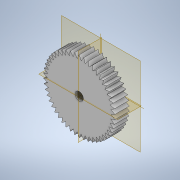
# Autodesk Inventor part: Zahnrad
Saved by Autodesk Inventor 2022 (Build 260153000, 153)
## iProperties
Created: 2022-05-06
Part Number: Zahnrad
Material: Generisch
Document SubType Name: Modeling
Designer: 123St
Density: 1 g/cm^3
Appearance: Vorgabe
Author: 123St
Autodesk Inventor part; units mm, degrees
sketch "Skizze1" plane through (0, 0, 0) normal (0, 0, 1) x (1, 0, 0)
  circle A0 centre (0, 0) radius 2.95
  circle A1 centre (0, 0) radius 5
  dimension "d0" = 5.9
  dimension "d1" = 10
  constraints: 2 centre point, 2 coincident
  measures "d0" diameter of A0
  measures "d1" diameter of A1
extrude "Extrusion1" add sketch "Skizze1" along normal blind 3
sketch "Skizze2" plane through (0, 0, 3) normal (0, 0, 1) x (1, 0, 0)
  circle A0 centre (0, 0) radius 15
  circle A1 centre (0, 0) radius 1.75
  dimension "d4" = 30
  dimension "d5" = 3.5
  constraints: 2 centre point, 2 coincident
  measures "d4" diameter of A0
  measures "d5" diameter of A1
extrude "Extrusion2" add sketch "Skizze2" along normal blind 6
sketch "Skizze3" plane through (0, 0, 9) normal (0, 0, 1) x (1, 0, 0)
  circle A0 centre (0, 0) radius 15 projected
  line L0 (0, 15) -> (-0.95, 13)
  line L1 (0, 15) -> (0.95, 13)
  line L2 (0, 21) -> (0, -21) projected
  line L3 (1.88, 14.8817) -> (0.6868, 13.0166)
  line L4 (1.88, 14.8817) -> (2.5718, 12.7784)
  line L5 (3.7303, 14.5287) -> (2.3128, 12.8278)
  line L6 (3.7303, 14.5287) -> (4.1531, 12.3553)
  line L7 (5.5219, 13.9466) -> (3.9023, 12.4368)
  line L8 (5.5219, 13.9466) -> (5.6689, 11.7374)
  line L9 (7.2263, 13.1446) -> (5.4303, 11.8497)
  line L10 (7.2263, 13.1446) -> (7.0953, 10.9343)
  line L11 (8.8168, 12.1353) -> (6.8726, 11.0756)
  line L12 (8.8168, 12.1353) -> (8.4098, 9.9588)
  line L13 (10.2682, 10.9345) -> (8.2066, 10.1269)
  line L14 (10.2682, 10.9345) -> (9.5916, 8.8263)
  line L15 (11.5577, 9.5614) -> (9.4111, 9.0185)
  line L16 (11.5577, 9.5614) -> (10.6222, 7.5545)
  line L17 (12.6649, 8.0374) -> (10.4672, 7.7679)
  line L18 (12.6649, 8.0374) -> (11.4853, 6.1636)
  line L19 (13.5724, 6.3867) -> (11.3583, 6.3947)
  line L20 (13.5724, 6.3867) -> (12.1672, 4.6755)
  line L21 (14.2658, 4.6353) -> (12.0702, 4.9207)
  line L22 (14.2658, 4.6353) -> (12.6573, 3.1137)
  line L23 (14.7343, 2.8107) -> (12.5917, 3.3691)
  line L24 (14.7343, 2.8107) -> (12.9477, 1.5028)
  line L25 (14.9704, 0.9419) -> (12.9147, 1.7644)
  line L26 (14.9704, 0.9419) -> (13.034, -0.1318)
  line L27 (14.9704, -0.9419) -> (13.034, 0.1318)
  line L28 (14.9704, -0.9419) -> (12.9147, -1.7644)
  line L29 (14.7343, -2.8107) -> (12.9477, -1.5028)
  line L30 (14.7343, -2.8107) -> (12.5917, -3.3691)
  line L31 (14.2658, -4.6353) -> (12.6573, -3.1137)
  line L32 (14.2658, -4.6353) -> (12.0702, -4.9207)
  line L33 (13.5724, -6.3867) -> (12.1672, -4.6755)
  line L34 (13.5724, -6.3867) -> (11.3583, -6.3947)
  line L35 (12.6649, -8.0374) -> (11.4853, -6.1636)
  line L36 (12.6649, -8.0374) -> (10.4672, -7.7679)
  line L37 (11.5577, -9.5614) -> (10.6222, -7.5545)
  line L38 (11.5577, -9.5614) -> (9.4111, -9.0185)
  line L39 (10.2682, -10.9345) -> (9.5916, -8.8263)
  line L40 (10.2682, -10.9345) -> (8.2066, -10.1269)
  line L41 (8.8168, -12.1353) -> (8.4098, -9.9588)
  line L42 (8.8168, -12.1353) -> (6.8726, -11.0756)
  line L43 (7.2263, -13.1446) -> (7.0953, -10.9343)
  line L44 (7.2263, -13.1446) -> (5.4303, -11.8497)
  line L45 (5.5219, -13.9466) -> (5.6689, -11.7374)
  line L46 (5.5219, -13.9466) -> (3.9023, -12.4368)
  line L47 (3.7303, -14.5287) -> (4.1531, -12.3553)
  line L48 (3.7303, -14.5287) -> (2.3128, -12.8278)
  line L49 (1.88, -14.8817) -> (2.5718, -12.7784)
  line L50 (1.88, -14.8817) -> (0.6868, -13.0166)
  line L51 (0, -15) -> (0.95, -13)
  line L52 (0, -15) -> (-0.95, -13)
  line L53 (-1.88, -14.8817) -> (-0.6868, -13.0166)
  line L54 (-1.88, -14.8817) -> (-2.5718, -12.7784)
  line L55 (-3.7303, -14.5287) -> (-2.3128, -12.8278)
  line L56 (-3.7303, -14.5287) -> (-4.1531, -12.3553)
  line L57 (-5.5219, -13.9466) -> (-3.9023, -12.4368)
  line L58 (-5.5219, -13.9466) -> (-5.6689, -11.7374)
  line L59 (-7.2263, -13.1446) -> (-5.4303, -11.8497)
  line L60 (-7.2263, -13.1446) -> (-7.0953, -10.9343)
  line L61 (-8.8168, -12.1353) -> (-6.8726, -11.0756)
  line L62 (-8.8168, -12.1353) -> (-8.4098, -9.9588)
  line L63 (-10.2682, -10.9345) -> (-8.2066, -10.1269)
  line L64 (-10.2682, -10.9345) -> (-9.5916, -8.8263)
  line L65 (-11.5577, -9.5614) -> (-9.4111, -9.0185)
  line L66 (-11.5577, -9.5614) -> (-10.6222, -7.5545)
  line L67 (-12.6649, -8.0374) -> (-10.4672, -7.7679)
  line L68 (-12.6649, -8.0374) -> (-11.4853, -6.1636)
  line L69 (-13.5724, -6.3867) -> (-11.3583, -6.3947)
  line L70 (-13.5724, -6.3867) -> (-12.1672, -4.6755)
  line L71 (-14.2658, -4.6353) -> (-12.0702, -4.9207)
  line L72 (-14.2658, -4.6353) -> (-12.6573, -3.1137)
  line L73 (-14.7343, -2.8107) -> (-12.5917, -3.3691)
  line L74 (-14.7343, -2.8107) -> (-12.9477, -1.5028)
  line L75 (-14.9704, -0.9419) -> (-12.9147, -1.7644)
  line L76 (-14.9704, -0.9419) -> (-13.034, 0.1318)
  line L77 (-14.9704, 0.9419) -> (-13.034, -0.1318)
  line L78 (-14.9704, 0.9419) -> (-12.9147, 1.7644)
  line L79 (-14.7343, 2.8107) -> (-12.9477, 1.5028)
  line L80 (-14.7343, 2.8107) -> (-12.5917, 3.3691)
  line L81 (-14.2658, 4.6353) -> (-12.6573, 3.1137)
  line L82 (-14.2658, 4.6353) -> (-12.0702, 4.9207)
  line L83 (-13.5724, 6.3867) -> (-12.1672, 4.6755)
  line L84 (-13.5724, 6.3867) -> (-11.3583, 6.3947)
  line L85 (-12.6649, 8.0374) -> (-11.4853, 6.1636)
  line L86 (-12.6649, 8.0374) -> (-10.4672, 7.7679)
  line L87 (-11.5577, 9.5614) -> (-10.6222, 7.5545)
  line L88 (-11.5577, 9.5614) -> (-9.4111, 9.0185)
  line L89 (-10.2682, 10.9345) -> (-9.5916, 8.8263)
  line L90 (-10.2682, 10.9345) -> (-8.2066, 10.1269)
  line L91 (-8.8168, 12.1353) -> (-8.4098, 9.9588)
  line L92 (-8.8168, 12.1353) -> (-6.8726, 11.0756)
  line L93 (-7.2263, 13.1446) -> (-7.0953, 10.9343)
  line L94 (-7.2263, 13.1446) -> (-5.4303, 11.8497)
  line L95 (-5.5219, 13.9466) -> (-5.6689, 11.7374)
  line L96 (-5.5219, 13.9466) -> (-3.9023, 12.4368)
  circle A1 centre (0, 0) radius 15
  line L97 (-3.7303, 14.5287) -> (-4.1531, 12.3553)
  line L98 (-3.7303, 14.5287) -> (-2.3128, 12.8278)
  line L99 (-1.88, 14.8817) -> (-2.5718, 12.7784)
  line L100 (-1.88, 14.8817) -> (-0.6868, 13.0166)
  point P0 (-4.1012, 12.6222)
  point P1 (-3.7303, 14.5287)
  point P2 (-3.7303, 14.5287)
  point P3 (-5.5219, 13.9466)
  point P4 (-5.6509, 12.0087)
  point P5 (-7.2263, 13.1446)
  point P6 (-7.2263, 13.1446)
  point P7 (-7.1114, 11.2057)
  point P8 (-8.4598, 10.2261)
  point P9 (-10.2682, 10.9345)
  point P10 (-10.2682, 10.9345)
  point P11 (-9.6747, 9.0852)
  point P12 (-11.5577, 9.5614)
  point P13 (-10.7371, 7.801)
  point P14 (-12.6649, 8.0374)
  point P15 (-12.6649, 8.0374)
  point P16 (-11.6302, 6.3937)
  point P17 (-12.3398, 4.8857)
  point P18 (-14.2658, 4.6353)
  point P19 (-12.8548, 3.3006)
  point P20 (-13.1671, 1.6634)
  point P21 (-14.9704, 0.9419)
  point P22 (-14.9704, 0.9419)
  point P23 (-13.2718, 0)
  point P24 (-14.9704, -0.9419)
  point P25 (-14.9704, -0.9419)
  point P26 (-13.1671, -1.6634)
  point P27 (-14.7343, -2.8107)
  point P28 (-14.7343, -2.8107)
  point P29 (-12.8548, -3.3006)
  point P30 (-14.2658, -4.6353)
  point P31 (-12.3398, -4.8857)
  point P32 (-13.5724, -6.3867)
  point P33 (-11.6302, -6.3937)
  point P34 (-12.6649, -8.0374)
  point P35 (-10.7371, -7.801)
  point P36 (-9.6747, -9.0852)
  point P37 (-10.2682, -10.9345)
  point P38 (-10.2682, -10.9345)
  point P39 (-8.4598, -10.2261)
  point P40 (-8.8168, -12.1353)
  point P41 (-7.1114, -11.2057)
  point P42 (-7.2263, -13.1446)
  point P43 (-7.2263, -13.1446)
  point P44 (-5.6509, -12.0087)
  point P45 (-5.5219, -13.9466)
  point P46 (-5.5219, -13.9466)
  point P47 (-4.1012, -12.6222)
  point P48 (-3.7303, -14.5287)
  point P49 (-2.4869, -13.0367)
  point P50 (-1.88, -14.8817)
  point P51 (-1.88, -14.8817)
  point P52 (-0.8333, -13.2456)
  point P53 (0, -15)
  point P54 (0, -15)
  point P55 (0.8333, -13.2456)
  point P56 (1.88, -14.8817)
  point P57 (1.88, -14.8817)
  point P58 (2.4869, -13.0367)
  point P59 (3.7303, -14.5287)
  point P60 (3.7303, -14.5287)
  point P61 (4.1012, -12.6222)
  point P62 (5.5219, -13.9466)
  point P63 (5.6509, -12.0087)
  point P64 (7.2263, -13.1446)
  point P65 (7.2263, -13.1446)
  point P66 (7.1114, -11.2057)
  point P67 (8.8168, -12.1353)
  point P68 (8.4598, -10.2261)
  point P69 (10.2682, -10.9345)
  point P70 (9.6747, -9.0852)
  point P71 (11.5577, -9.5614)
  point P72 (10.7371, -7.801)
  point P73 (12.6649, -8.0374)
  point P74 (11.6302, -6.3937)
  point P75 (13.5724, -6.3867)
  point P76 (12.3398, -4.8857)
  point P77 (14.2658, -4.6353)
  point P78 (12.8548, -3.3006)
  point P79 (14.7343, -2.8107)
  point P80 (14.7343, -2.8107)
  point P81 (13.1671, -1.6634)
  point P82 (14.9704, -0.9419)
  point P83 (14.9704, -0.9419)
  point P84 (13.2718, 0)
  point P85 (14.9704, 0.9419)
  point P86 (13.1671, 1.6634)
  point P87 (14.7343, 2.8107)
  point P88 (12.8548, 3.3006)
  point P89 (14.2658, 4.6353)
  point P90 (14.2658, 4.6353)
  point P91 (12.3398, 4.8857)
  point P92 (13.5724, 6.3867)
  point P93 (13.5724, 6.3867)
  point P94 (11.6302, 6.3937)
  point P95 (12.6649, 8.0374)
  point P96 (12.6649, 8.0374)
  point P97 (10.7371, 7.801)
  point P98 (11.5577, 9.5614)
  point P99 (9.6747, 9.0852)
  point P100 (10.2682, 10.9345)
  point P101 (10.2682, 10.9345)
  point P102 (8.4598, 10.2261)
  point P103 (7.1114, 11.2057)
  point P104 (7.2263, 13.1446)
  point P105 (7.2263, 13.1446)
  point P106 (5.6509, 12.0087)
  point P107 (5.5219, 13.9466)
  point P108 (5.5219, 13.9466)
  point P109 (4.1012, 12.6222)
  point P110 (3.7303, 14.5287)
  point P111 (3.7303, 14.5287)
  point P112 (2.4869, 13.0367)
  point P113 (1.88, 14.8817)
  point P114 (1.88, 14.8817)
  point P115 (0.8333, 13.2456)
  point P116 (-0.8366, 13.0314)
  point P117 (-2.4869, 13.0367)
  point P118 (-0.8333, 13.2456)
  dimension "d12" = 1.9
  dimension "d13" = 0.95
  dimension "d14" = 0
  dimension "d15" = 2
  dimension "d16" = 2
  dimension "d17" = 15
  dimension "d20" = 360
  constraints: 200 end point, 3 coincident, 1 centre point, 299 other
  measures "d12" distance of L0.end L1.end
  measures "d13" distance from line of L2 L1.end
  measures "d14" horizontal distance of point (0, 0) L0.start
  measures "d15" vertical distance of L0.end L0.start
  measures "d16" vertical distance of L0.start L1.end
  measures "d17" distance of point (0, 0) L0.start
extrude "Extrusion3" cut sketch "Skizze3" against normal blind 6 contours A0 L27 L26 | L25 L24 A0 | A0 L29 L28 | L23 L22 A0 | A0 L31 L30 | L21 L20 A0 | A0 L33 L32 | L19 L18 A0 | A0 L35 L34 | L17 L16 A0 | A0 L37 L36 | L15 L14 A0 | A0 L39 L38 | L13 L12 A0 | A0 L41 L40 | L11 L10 A0 | A0 L43 L42 | L9 L8 A0 | A0 L45 L44 | L7 L6 A0 | A0 L47 L46 | L5 L4 A0 | A0 L49 L48 | L3 L1 A0 | A0 L51 L50 | L0 L100 A0 | A0 L53 L52 | L99 L98 A0 | A0 L55 L54 | L97 L96 A0 | A0 L57 L56 | L95 L94 A0 | A0 L59 L58 | L93 L92 A0 | A0 L61 L60 | L91 L90 A0 | A0 L63 L62 | L89 L88 A0 | A0 L65 L64 | L87 L86 A0 | A0 L67 L66 | L85 L84 A0 | A0 L69 L68 | L83 L82 A0 | A0 L71 L70 | L81 L80 A0 | A0 L73 L72 | L79 L78 A0 | A0 L75 L74 | L77 L76 A0
fillet "Rundung1" [suppressed]
sketch "Skizze4" plane through (0, 0, 3) normal (0, 0, -1) x (-1, 0, 0)
  circle A0 centre (0, 0) radius 2.95
  constraints: 1 centre point, 1 coincident
extrude "Extrusion4" cut sketch "Skizze4" against normal blind 1
equation "\"d13\" = 0.5 * d12"
